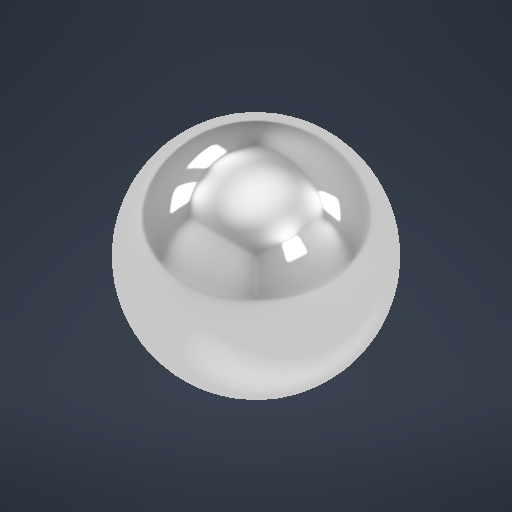
# Autodesk Inventor part: 2.5mm_BALL_BEARINGS
Saved by Autodesk Inventor 2026.2 (Build 302298010, 298A)
## iProperties
Created: 2026-03-05
Part Number: 2.5mm_BALL_BEARINGS
Material: Steel, O1, HT 58-60 Rc
Document SubType Name: Modeling
Designer: 4aida
Density: 7.86 g/cm^3
Appearance: Chrome - Polished
Author: 4aida
Autodesk Inventor part; units mm, degrees
ref_plane "YZ Plane" through (0, 0, 0) normal (1, 0, 0) x (0, 1, 0)
ref_plane "XZ Plane" through (0, 0, 0) normal (0, 1, 0) x (-1, 0, 0)
ref_plane "XY Plane" through (0, 0, 0) normal (0, 0, 1) x (1, 0, 0)
sketch "Sketch1" plane through (0, 0, 0) normal (1, 0, 0) x (0, 1, 0)
  arc A0 (1.25, 0) -> (-1.25, 0) centre (0, 0) ccw
  line L0 (1.25, 0) -> (-1.25, 0)
  dimension "d0" = 1.25
  constraints: 2 coincident, 2 end point, 2 point on circle, 1 centre point, 1 horizontal, 1 midpoint
  measures "d0" radius of A0
revolve "Revolution1" add sketch "Sketch1" angle 360 about axis through (0, 1.25, 0) along (0, -1, 0)
body "Solid1"
